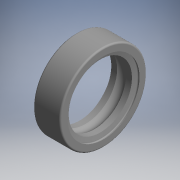
# Autodesk Inventor part: SKF_634-2Z_PART2
Saved by Autodesk Inventor 2017.3 (Build 213256000, 256)
## iProperties
Part Number: SKF_634-2Z_PART2
Material: Generic
Catalog Web Link: www.cadenas.de
Description: -Deep groove ball bearings
Vendor: SKF
Document SubType Name: Modeling
Designer: partserver
Manufacturer: SKF
Mass: 5 g
Surface Area: 6.31504 cm^2
Volume: 0.414203 cm^3
Density: 1 g/cm^3
Appearance: PSOLRGB-175-175-175
Category: PARTsolutions
Company: SKF
Title: SKF_634-2Z_PART2
Author: Cadenas PARTsolutions
Comments: Deep groove ball bearings
PSOL_IDENT_0: {$CADENAS_DATA\23d-libs\skf\bearings_units_and_housings\ball_bearings\deep_groove_ball_bearings\bb1_
PSOL_IDENT_1: 001_101.prj},199 {VTYP=3D},{NB=SKF_634-2Z_PART2},{LINA=SKF_634-2Z_PART2},{NN=BB1_001_101_PART2},{NOP
PSOL_IDENT_2: RJ=TRUE},{DATE=11.06.2021 05:15:49},{GEOMDATE=07.06.2021 05:44:42},{VERSION=},{LINEID=14700},{WBVAR=
PSOL_IDENT_3: },{WBNUMERIC=}  {NB=SKF_634-2Z_PART2},{LINA=SKF_634-2Z_PART2},{KT=DUMMY},{DESIGNATION=634-2Z},{R12=0
PSOL_IDENT_4: .30},{DD=4.000},{D=16.000},{B=5.000},{C=},{CX=},{CXX=},{CA=0.000},{XXVARIANT=},{XXDESIGN=Single row}
PSOL_IDENT_5: ,{XXSEALING=Shield on both sides},{DESIGN=dgbbz},{DESIGNIR=dgbbz},{VARIANT=},{DD1=8.40},{DD2=},{DD2X=
PSOL_IDENT_6: },{DD2A=0.00},{D1=11.70},{D1X=MIN},{D2=13.3},{D2A=13.30},{D3=},{D3X=},{D3A=0.000},{D4=},{HH=MIN},{BB=
PSOL_IDENT_7: MIN},{BBX=},{BBA=0.000},{FF=},{R0MAX=MIN},{R0=MIN},{PITCH=10.00},{DW=2.381},{DDAMIN=6.400},{DDAMAX=8
PSOL_IDENT_8: .300},{DDBMIN=MIN},{DDBMAX=MIN},{DBMIN=MIN},{DAMAX=13.600},{BBAMIN=MIN},{CAMAX=MIN},{RAMAX=0.300},{L
PSOL_IDENT_9: OAD1=1.110},{LOAD2=0.380},{LOAD3=0.016},{SPEED1=95000},{SPEED2=48000},{KR=0.030},{F0=8.400},{Z=7},{I
PSOL_IDENT_10: I=1},{MASS=0.005},{BEARING=634-2Z},{RING=},{HELP=2.150},{HELP2=1.350},{DD1ALG=4.200},{YALG=4.200},{P
PSOL_IDENT_11: ITCH1=10.000},{DW1=2.381},{YALG1=5.850},{HALG1=2.150},{SH=4.200},{CU=0.524},{HALG=2.2},{B1=0},{SHIEL
PSOL_IDENT_12: DHELP=2},{D4A=0.000},{FFA=0.000},{RS1=}
NB: SKF_634-2Z_PART2
NT: Deep groove ball bearings
NBSYN: SKF_$DESIGNATION._PART2
LINA: SKF_634-2Z_PART2
CATALOG: SKF
DESIGNATION: 634-2Z
R12: 0.3
DD: 4
D: 16
B: 5
D2: 13.3
LOAD1: 1.11
LOAD2: 0.38
LOAD3: 0.016
SPEED1: 95000
SPEED2: 48000
BEARING: 634-2Z
SUPPLIER: SKF
ARTICLENO: SKF_634-2Z_PART2
BOMINFO: SKF_634-2Z_PART2
CREATOR: CADENAS GmbH
Autodesk Inventor part; units mm, degrees
ref_plane "YZ Plane" through (0, 0, 0) normal (1, 0, 0) x (0, 1, 0)
ref_plane "XZ Plane" through (0, 0, 0) normal (0, 1, 0) x (-1, 0, 0)
ref_plane "XY Plane" through (0, 0, 0) normal (0, 0, 1) x (1, 0, 0)
sketch "Sketch_22" plane through (0, 0, 0) normal (0, 0, 1) x (1, 0, 0)
  line L0 (50, 0) -> (-50, 0)
  line L1 (0, 6.65) -> (0.09, 6.65)
  arc A0 (0.45, 6.65) -> (0.09, 6.65) centre (0.27, 6.65) ccw
  line L2 (0.45, 6.65) -> (0.5911, 5.85)
  line L3 (0.5911, 5.85) -> (1.6665, 5.85)
  arc A1 (3.3335, 5.85) -> (1.6665, 5.85) centre (2.5, 5) ccw
  line L4 (3.3335, 5.85) -> (4.4089, 5.85)
  line L5 (4.4089, 5.85) -> (4.55, 6.65)
  arc A2 (4.91, 6.65) -> (4.55, 6.65) centre (4.73, 6.65) ccw
  line L6 (4.91, 6.65) -> (5, 6.65)
  line L7 (5, 6.65) -> (5, 7.7)
  arc A3 (5, 7.7) -> (4.7, 8) centre (4.7, 7.7) ccw
  line L8 (4.7, 8) -> (0.3, 8)
  arc A4 (0.3, 8) -> (0, 7.7) centre (0.3, 7.7) ccw
  line L9 (0, 7.7) -> (0, 6.65)
  constraints: 20 end point, 10 point on circle, 5 centre point
revolve "Revolution1" add sketch "Sketch_22" angle 360 about axis through (50, 0, 0) along (1, 0, 0)
body "Solid1"
